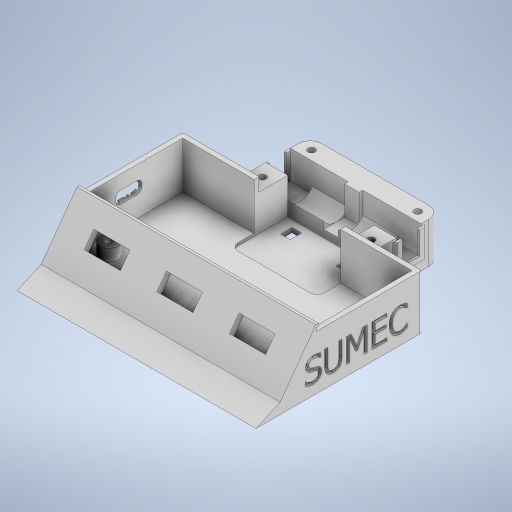
# Autodesk Inventor part: Sumec_telo_V4.1
Saved by Autodesk Inventor 2023 (Build 270158000, 158)
## iProperties
Created: 2023-03-18
Part Number: Sumec_telo_V4.1
Material: Všeobecné
Document SubType Name: Modeling
Designer: jaryj
Density: 1 g/cm^3
Appearance: Výchozí
Author: jaryj
Autodesk Inventor part; units mm, degrees
ref_plane "YZ Plane" through (0, 0, 0) normal (1, 0, 0) x (0, 1, 0)
ref_plane "XZ Plane" through (0, 0, 0) normal (0, 1, 0) x (-1, 0, 0)
ref_plane "XY Plane" through (0, 0, 0) normal (0, 0, 1) x (1, 0, 0)
sketch "Náčrt1" plane through (0, 0, 0) normal (0, 1, 0) x (-1, 0, 0)
  line L0 (0, 0) -> (49.75, 0)
  line L1 (49.75, 0) -> (49.75, -69)
  line L2 (49.75, -69) -> (18, -69)
  line L3 (18, -69) -> (18, -81)
  line L4 (18, -81) -> (27.25, -81)
  line L5 (27.25, -81) -> (27.25, -69)
  line L6 (27.25, -81) -> (27.25, -91.25)
  line L7 (27.25, -91.25) -> (27.25, -99.5)
  line L8 (27.25, -99.5) -> (0, -99.5)
  line L9 (0, -99.5) -> (0, -91.25)
  line L10 (0, -91.25) -> (27.25, -91.25)
  line L11 (0, -91.25) -> (0, -81)
  line L12 (0, -81) -> (18, -81)
  line L13 (0, -81) -> (0, 0)
  line L14 (18, -69) -> (18, -57.25)
  line L15 (18, -57.25) -> (0, -57.25)
  line L16 (47.75, -25) -> (47.75, -67)
  line L17 (47.75, -67) -> (18, -67)
  line L18 (0, -25) -> (47.75, -25)
  dimension "d0" = 49.75
  dimension "d1" = 69
  dimension "d2" = 12
  dimension "d3" = 10.25
  dimension "d4" = 8.25
  dimension "d5" = 27.25
  dimension "d6" = 18
  dimension "d9" = 2
  dimension "d13" = 25
  dimension "d18" = 2
  dimension "d190" = 9.75
  constraints: 38 end point, 12 perpendicular, 7 point on line, 1 horizontal, 1 vertical
  measures "d0" distance of L0.start L0.end
  measures "d1" distance of L0.end L1.end
  measures "d2" distance of L4.end L5.end
  measures "d3" distance of L4.end L6.end
  measures "d4" distance of L6.end L7.end
  measures "d5" distance of L7.end L8.end
  measures "d6" distance of L3.end L11.end
  measures "d9" distance between parallel lines of L17 L2
  measures "d13" distance between parallel lines of L0 L18
  measures "d18" distance between parallel lines of L1 L16
  measures "d190" distance between parallel lines of L17 L15
extrude "Vysunutí1" add sketch "Náčrt1" along normal blind 3 contours L18 L16 L17 L14 L15 L13
extrude "Vysunutí2" add sketch "Náčrt1" along normal blind 1.888 contours L15 L14 L3 L12 L13
extrude "Vysunutí3" add sketch "Náčrt1" along normal blind 22.5 contours L0 L1 L2 L14 L17 L16 L18 L13
extrude "Vysunutí4" add sketch "Náčrt1" along normal blind 17 contours L5 L4 L3 L2 | L10 L7 L8 L9
extrude "Vysunutí15" add sketch "Náčrt1" along normal blind 5 contours L12 L4 L6 L10 L11
sketch "Náčrt2" plane through (-49.75, 0, -69) normal (-1, 0, 0) x (0, 0, 1)
  line L0 (69, 0) -> (69, 22.5) projected
  line L1 (69, 0) -> (59, 4.5)
  line L2 (0, 0) -> (69, 0) projected
  line L3 (44, 0) -> (44, 22.5)
  line L4 (44, 3) -> (44, 22.5) projected
  line L5 (44, 22.5) -> (44, 25)
  line L6 (44, 25) -> (59, 4.5)
  line L7 (0, 22.5) -> (69, 22.5) projected
  point P0 (45.8293, 22.5)
  dimension "d23" = 25
  dimension "d24" = 4.5
  dimension "d25" = 10
  constraints: 8 end point, 2 point on line, 1 vertical
  measures "d23" distance of L3.start L5.end
  measures "d24" distance from line of L2 L1.end
  measures "d25" horizontal distance of L0.start L1.end
extrude "Vysunutí5" cut sketch "Náčrt2" against normal through all contours L1 L6 L7 L0
extrude "Vysunutí6" add sketch "Náčrt2" against normal up to surface (49.75 mm away) contours L7 L5 L6
sketch "Náčrt3" plane through (0, 3, -25) normal (0, 0, -1) x (-1, 0, 0)
  line L0 (22.75, 15.167) -> (37.75, 15.167)
  line L1 (37.75, 15.167) -> (37.75, 0)
  line L2 (37.75, 0) -> (22.75, 0)
  line L3 (22.75, 0) -> (22.75, 15.167)
  line L4 (0, 15.167) -> (7.5, 15.167)
  line L5 (7.5, 15.167) -> (7.5, 0)
  line L6 (7.5, 0) -> (0, 0)
  line L7 (0, 0) -> (0, 15.167)
  line L8 (49.75, -3) -> (0, -3) projected
  dimension "d30" = 15
  dimension "d31" = 7.5
  dimension "d32" = 15.167
  dimension "d33" = 3
  dimension "d34" = 15.25
  constraints: 16 end point, 4 perpendicular, 4 point on line, 1 horizontal, 1 vertical alignment
  measures "d30" distance of L0.start L0.end
  measures "d31" distance of L4.start L4.end
  measures "d32" distance of L0.end L1.end
  measures "d33" distance between parallel lines of L8 L6
  measures "d34" distance between parallel lines of L3 L5
extrude "Vysunutí7" cut sketch "Náčrt3" against normal blind 9
sketch "Náčrt7" plane through (-47.75, 3, -67) normal (1, 0, 0) x (0, 0, -1)
  line L0 (-57, 1.5) -> (-42, 22) projected
  line L1 (-42, 15.167) -> (-42, 0) projected
  line L2 (-42, 0) -> (-50, 0)
  line L3 (-42, 0) -> (-51, 0) projected
  line L4 (-50, 0) -> (-50, 6.833)
  line L5 (-50, 6.833) -> (-42, 17.7664)
  line L6 (-42, 17.7664) -> (-42, 0)
  point P0 (-67, -3)
  point P1 (-42, 22)
  point P2 (-38.3293, 19.5)
  point P3 (-36.5, 2)
  point P4 (-36.5, 2)
  dimension "d45" = 8
  dimension "d46" = 2.5
  constraints: 8 end point, 2 perpendicular, 1 collinear, 2 other
  measures "d45" distance of L2.start L2.end
extrude "Vysunutí9" cut sketch "Náčrt7" along normal through all
sketch "Náčrt13" plane through (0, 17, 0) normal (0, 1, 0) x (1, 0, 0)
  line L0 (-18, 81) -> (-27.25, 81) projected
  line L1 (-27.25, 81) -> (-27.25, 69) projected
  point P0 (0, 0)
  point P1 (-22.625, 75)
  dimension "d84" = 6
  dimension "d85" = 4.625
  measures "d84" distance from line of L0 point (-22.625, 75)
  measures "d85" distance from line of L1 point (-22.625, 75)
hole "Díra2" at (-22.625, 17, -75) direction (0, -1, 0) diameter 3 depth 6
sketch "Náčrt14" plane through (0, 17, 0) normal (0, 1, 0) x (1, 0, 0)
  line L0 (-27.25, 99.5) -> (-27.25, 91.25) projected
  line L1 (0, 99.5) -> (-27.25, 99.5) projected
  point P0 (0, 0)
  point P1 (-22.125, 95)
  dimension "d93" = 5.125
  dimension "d101" = 4.5
  measures "d93" distance from line of L0 point (-22.125, 95)
  measures "d101" distance from line of L1 point (-22.125, 95)
hole "Díra3" at (-22.125, 17, -95) direction (0, -1, 0) diameter 3 depth 6
fillet "Zaoblení1" radius 3 1 edges at (-18, 2.444, -57.25)
fillet "Zaoblení2" radius 1 1 edges at (-49.75, 11.25, -69)
fillet "Zaoblení3" radius 5 1 edges at (-27.25, 8.5, -99.5)
sketch "Náčrt24" plane through (-18, 3, -67) normal (1, 0, 0) x (0, 0, -1)
  line L0 (24.25, 2) -> (24.25, 14) projected
  line L1 (24.25, 2) -> (14, 2) projected
  line L2 (14, 2) -> (14, 14) projected
  line L3 (14, 2) -> (24.25, 2) projected
  line L4 (24.25, 4.88) -> (24.25, 2)
  line L5 (24.25, 2) -> (14, 2)
  line L6 (14, 2) -> (14, 4.88)
  arc A0 (14, 4.88) -> (24.25, 4.88) centre (19.125, 8) ccw
  point P0 (-67, -3)
  point P1 (19.125, 2)
  dimension "d200" = 6
  constraints: 6 end point, 2 perpendicular, 2 point on circle, 2 point on line, 1 centre point, 1 horizontal alignment, 1 tangent
  measures "d200" radius of A0
extrude "Vysunutí22" add sketch "Náčrt24" along normal blind 15
sketch "Náčrt21" plane through (-27.25, 0, -69) normal (-1, 0, 0) x (0, 0, 1)
  line L0 (-20.75, 16) -> (-23.75, 16)
  line L1 (-22.25, 17) -> (-30.5, 17) projected
  line L2 (-23.75, 3.5) -> (-10.5, 3.5)
  line L3 (-10.5, 3.5) -> (-10.5, 16)
  line L4 (-10.5, 16) -> (-13.5, 16)
  line L5 (-13.5, 16) -> (-13.5, 6.5)
  line L6 (-13.5, 6.5) -> (-20.75, 6.5)
  line L7 (-20.75, 6.5) -> (-20.75, 16)
  line L8 (-23.75, 16) -> (-23.75, 3.5)
  line L9 (-22.25, 5) -> (-22.25, 17) projected
  line L10 (-22.25, 5) -> (-12, 5) projected
  line L11 (-12, 5) -> (-12, 17) projected
  line L12 (-12, 17) -> (0, 17) projected
  point P0 (69, 0)
  dimension "d172" = 1.5
  dimension "d173" = 1.5
  dimension "d174" = 1.5
  dimension "d175" = 1.5
  dimension "d176" = 1.5
  dimension "d177" = 1.5
  dimension "d180" = 1
  constraints: 12 end point, 3 perpendicular, 1 horizontal, 1 parallel, 1 vertical, 8 other
  measures "d172" distance between parallel lines of L7 L9
  measures "d173" distance between parallel lines of L6 L10
  measures "d174" distance between parallel lines of L5 L11
  measures "d175" distance between parallel lines of L11 L3
  measures "d176" distance between parallel lines of L2 L10
  measures "d177" distance between parallel lines of L8 L9
extrude "Vysunutí19" add sketch "Náčrt21" along normal blind 1
chamfer "Zkosení1" distance 1 angle 45 3 edges at (-28.25, 9.75, -92.75) (-28.25, 3.5, -86.125) (-28.25, 9.75, -79.5)
sketch "Náčrt27" plane through (-49.75, 22.5, -25) normal (-1, 0, 0) x (0, 0, 1)
  line L0 (0, 2.5) -> (0, 0) projected
  line L1 (0, 2.5) -> (-1, 2.5)
  line L2 (-1, 2.5) -> (-1, 1.5)
  line L3 (-1, 1.5) -> (0, 1.5)
  line L4 (0, 1.5) -> (0, 2.5)
  point P0 (25, -22.5)
  point P1 (0, 1.5)
  dimension "d219" = 1
  dimension "d220" = 1
  constraints: 8 end point, 2 parallel, 1 horizontal, 1 perpendicular
  measures "d219" distance of L2.end L3.end
  measures "d220" distance of L1.end L2.end
extrude "Vysunutí25" add sketch "Náčrt27" against normal up to surface (49.75 mm away)
mirror "Zrcadlit1" about plane through (0, 0, -25) normal (1, 0, 0)
sketch "Náčrt16" plane through (0, 1.888, 0) normal (0, 1, 0) x (1, 0, 0)
  line L0 (-9.4, 73.375) -> (-13.4, 73.375)
  line L1 (-13.4, 73.375) -> (-13.4, 78.125)
  line L2 (-13.4, 78.125) -> (-9.4, 78.125)
  line L3 (-9.4, 78.125) -> (-9.4, 73.375)
  line L4 (-18, 69) -> (-18, 81) projected
  line L5 (13.75, 73.375) -> (9.75, 73.375)
  line L6 (9.75, 73.375) -> (9.75, 78.125)
  line L7 (9.75, 78.125) -> (13.75, 78.125)
  line L8 (13.75, 78.125) -> (13.75, 73.375)
  line L9 (18, 69) -> (18, 81) projected
  line L10 (-18, 81) -> (18, 81) projected
  point P0 (0, 0)
  dimension "d128" = 4
  dimension "d129" = 4.75
  dimension "d130" = 4.6
  dimension "d134" = 4.25
  dimension "d192" = 2.875
  constraints: 16 end point, 4 parallel, 2 equal length, 2 perpendicular, 1 horizontal, 1 horizontal alignment
  measures "d128" distance of L0.start L0.end
  measures "d129" distance of L2.end L0.start
  measures "d130" distance between parallel lines of L4 L1
  measures "d134" distance between parallel lines of L9 L8
  measures "d192" distance between parallel lines of L10 L2
extrude "Vysunutí16" cut sketch "Náčrt16" against normal through all
sketch "Náčrt17" plane through (0, 3, 0) normal (0, 1, 0) x (1, 0, 0)
  line L0 (-47.75, 17) -> (-37.75, 17) projected
  line L1 (-47.75, 17) -> (-47.75, 67) projected
  line L2 (47.75, 17) -> (37.75, 17) projected
  line L3 (47.75, 17) -> (47.75, 67) projected
  line L4 (-39.4, 19.625) -> (-43.4, 19.625)
  line L5 (-43.4, 19.625) -> (-43.4, 24.375)
  line L6 (-43.4, 24.375) -> (-39.4, 24.375)
  line L7 (-39.4, 24.375) -> (-39.4, 19.625)
  line L8 (42.75, 19.625) -> (38.75, 19.625)
  line L9 (38.75, 19.625) -> (38.75, 24.375)
  line L10 (38.75, 24.375) -> (42.75, 24.375)
  line L11 (42.75, 24.375) -> (42.75, 19.625)
  point P0 (0, 0)
  point P1 (-48, 67)
  point P2 (48, 67)
  point P3 (-41.4, 19.625)
  point P4 (40.75, 19.625)
  point P5 (-47.75, 67)
  point P6 (47.75, 67)
  dimension "d137" = 4
  dimension "d138" = 4.75
  dimension "d139" = 4.35
  dimension "d143" = 2.625
  dimension "d144" = 5
  dimension "d146" = 2.625
  constraints: 16 end point, 4 parallel, 2 equal length, 2 horizontal, 2 midpoint, 2 perpendicular, 2 other
  measures "d137" distance of L4.start L4.end
  measures "d138" distance of L6.end L4.start
  measures "d143" distance between parallel lines of L0 L4
  measures "d146" distance from line of L2 point (40.75, 19.625)
extrude "Vysunutí17" cut sketch "Náčrt17" against normal through all
sketch "Náčrt18" plane through (0, 3, 0) normal (0, 1, 0) x (1, 0, 0)
  circle A0 centre (39.25, 59) radius 3.75
  circle A1 centre (-40.5, 29) radius 3.75
  line L0 (47.75, 67) -> (18, 67) projected
  line L1 (47.75, 25) -> (47.75, 67) projected
  line L2 (-47.75, 17) -> (-37.75, 17) projected
  line L3 (-47.75, 17) -> (-47.75, 67) projected
  point P0 (0, 0)
  point P1 (42.5, 67)
  point P2 (-48, 67)
  point P3 (-47.75, 67)
  dimension "d149" = 7.5
  dimension "d150" = 8
  dimension "d151" = 8.5
  dimension "d152" = 12
  dimension "d153" = 7.25
  constraints: 2 centre point, 1 equal radius, 1 other
  measures "d149" diameter of A0
  measures "d150" distance from line of A0.centre L0
  measures "d151" distance from line of L1 A0.centre
  measures "d152" distance from line of L2 A1.centre
extrude "Vysunutí18" add sketch "Náčrt18" along normal blind 5
sketch "Náčrt19" plane through (39.25, 8, -59) normal (0, 1, 0) x (1, 0, 0)
  circle A0 centre (0, 0) radius 3.75 projected
  point P0 (-39.25, -59)
  constraints: 1 coincident
hole "Díra4" at (39.25, 8, -59) direction (0, -1, 0) diameter 3 depth 6
sketch "Náčrt20" plane through (-40.5, 8, -29) normal (0, 1, 0) x (1, 0, 0)
  circle A0 centre (0, 0) radius 3.75 projected
  point P0 (40.5, -29)
  constraints: 1 coincident
hole "Díra5" at (-40.5, 8, -29) direction (0, -1, 0) diameter 3 depth 6
sketch "Náčrt25" plane through (-18, 7.88, -91.25) normal (0, 0, 1) x (1, 0, 0)
  line L0 (-4.25, 9.12) -> (40.25, 9.12) projected
  line L1 (15, 9.12) -> (21, 9.12)
  line L2 (21, 9.12) -> (21, -2.88)
  line L3 (21, -2.88) -> (15, -2.88)
  line L4 (15, -2.88) -> (15, 9.12)
  line L5 (15, 0) -> (15, -2.88) projected
  line L6 (21, 0) -> (21, -2.88) projected
  point P0 (18, -7.88)
  dimension "d203" = 12
  dimension "d204" = 6
  constraints: 8 end point, 2 parallel, 1 coincident, 1 horizontal, 1 perpendicular, 1 point on line
  measures "d203" distance of L3.end L1.start
  measures "d204" distance between parallel lines of L2 L4
extrude "Vysunutí23" add sketch "Náčrt25" along normal blind 1.5
sketch "Náčrt26" plane through (-49.75, 0, -68) normal (-1, 0, 0) x (0, 0, 1)
  line L0 (20, 11.7) -> (27, 11.7)
  line L1 (27, 16.7) -> (20, 16.7)
  line L2 (18, 14.7) -> (18, 13.7)
  line L3 (29, 14.7) -> (29, 13.7)
  line L4 (0, 0) -> (68, 0) projected
  line L5 (0, 0) -> (0, 22.5) projected
  arc A0 (20, 16.7) -> (18, 14.7) centre (20, 14.7) ccw
  arc A1 (18, 13.7) -> (20, 11.7) centre (20, 13.7) ccw
  arc A2 (29, 14.7) -> (27, 16.7) centre (27, 14.7) ccw
  arc A3 (27, 11.7) -> (29, 13.7) centre (27, 13.7) ccw
  dimension "d207" = 11.7
  dimension "d208" = 5
  dimension "d209" = 11
  dimension "d210" = 18
  dimension "d211" = 2
  constraints: 8 end point, 8 point on circle, 8 tangent, 4 centre point, 3 equal radius, 1 horizontal, 1 parallel, 1 vertical
  measures "d207" distance between parallel lines of L4 L0
  measures "d208" distance between parallel lines of L0 L1
  measures "d209" distance between parallel lines of L3 L2
  measures "d210" distance between parallel lines of L5 L2
  measures "d211" radius of A0
extrude "Vysunutí24" cut sketch "Náčrt26" against normal up to surface (2 mm away)
sketch "Náčrt28" plane through (49.75, 0, 0) normal (1, 0, 0) x (0, 0, -1)
  line L0 (20, 14.5) -> (64, 14.5) construction
  line L1 (64, 14.5) -> (64, 4) construction
  line L2 (64, 4) -> (20, 4) construction
  line L3 (20, 4) -> (20, 14.5) construction
  line L4 (68, 22.5) -> (25, 22.5) projected
  line L5 (68, 0) -> (68, 22.5) projected
  spline S0 degree 2 poles (23.8006, 4.1434) (22.7147, 4.1434) (21.1912, 4.5972) (20.5186, 4.9214) knots 0 0 0 1 2 2 2
  line L6 (20.5186, 4.9214) -> (20.5186, 6.5908)
  line L7 (20.5186, 6.5908) -> (20.6159, 6.5908)
  spline S1 degree 2 poles (20.6159, 6.5908) (21.2723, 5.9749) (22.9335, 5.2942) (23.7034, 5.2942) knots 0 0 0 1 2 2 2
  spline S2 degree 2 poles (23.7034, 5.2942) (24.8055, 5.2942) (25.9319, 6.2099) (25.9319, 6.9635) knots 0 0 0 1 2 2 2
  spline S3 degree 2 poles (25.9319, 6.9635) (25.9319, 7.5632) (25.3404, 8.3088) (24.7002, 8.4951) knots 0 0 0 1 2 2 2
  spline S4 degree 2 poles (24.7002, 8.4951) (24.2382, 8.6248) (23.4684, 8.8031) (22.893, 8.9489) knots 0 0 0 1 2 2 2
  spline S5 degree 2 poles (22.893, 8.9489) (22.3744, 9.0867) (21.5559, 9.5) (21.2399, 9.8323) knots 0 0 0 1 2 2 2
  spline S6 degree 2 poles (21.2399, 9.8323) (20.9319, 10.1645) (20.5916, 11.0559) (20.5916, 11.6394) knots 0 0 0 1 2 2 2
  spline S7 degree 2 poles (20.5916, 11.6394) (20.5916, 12.8549) (22.4878, 14.5) (23.9546, 14.5) knots 0 0 0 1 2 2 2
  spline S8 degree 2 poles (23.9546, 14.5) (24.7974, 14.5) (26.2885, 14.1677) (26.9287, 13.8517) knots 0 0 0 1 2 2 2
  line L8 (26.9287, 13.8517) -> (26.9287, 12.2634)
  line L9 (26.9287, 12.2634) -> (26.8314, 12.2634)
  spline S9 degree 2 poles (26.8314, 12.2634) (26.3533, 12.701) (24.8622, 13.3493) (24.0438, 13.3493) knots 0 0 0 1 2 2 2
  spline S10 degree 2 poles (24.0438, 13.3493) (23.1199, 13.3493) (21.9773, 12.4822) (21.9773, 11.7771) knots 0 0 0 1 2 2 2
  spline S11 degree 2 poles (21.9773, 11.7771) (21.9773, 11.1451) (22.6499, 10.3914) (23.282, 10.2212) knots 0 0 0 1 2 2 2
  spline S12 degree 2 poles (23.282, 10.2212) (23.7034, 10.1078) (24.9271, 9.816) (25.3323, 9.6945) knots 0 0 0 1 2 2 2
  spline S13 degree 2 poles (25.3323, 9.6945) (26.3614, 9.3784) (27.3177, 8.1062) (27.3177, 7.1742) knots 0 0 0 1 2 2 2
  spline S14 degree 2 poles (27.3177, 7.1742) (27.3177, 6.5827) (26.8395, 5.4481) (26.41, 5.0511) knots 0 0 0 1 2 2 2
  spline S15 degree 2 poles (26.41, 5.0511) (25.9319, 4.6135) (24.7164, 4.1434) (23.8006, 4.1434) knots 0 0 0 1 2 2 2
  spline S16 degree 2 poles (32.1637, 4.111) (31.2804, 4.111) (29.9676, 4.5729) (29.5057, 5.0348) knots 0 0 0 1 2 2 2
  spline S17 degree 2 poles (29.5057, 5.0348) (28.9789, 5.5535) (28.5494, 7.0122) (28.5494, 8.0818) knots 0 0 0 1 2 2 2
  line L10 (28.5494, 8.0818) -> (28.5494, 14.3217)
  line L11 (28.5494, 14.3217) -> (29.8784, 14.3217)
  line L12 (29.8784, 14.3217) -> (29.8784, 8.0818)
  spline S18 degree 2 poles (29.8784, 8.0818) (29.8784, 7.3849) (30.0567, 6.4449) (30.3079, 6.064) knots 0 0 0 1 2 2 2
  spline S19 degree 2 poles (30.3079, 6.064) (30.5754, 5.6588) (31.4992, 5.2455) (32.1637, 5.2455) knots 0 0 0 1 2 2 2
  spline S20 degree 2 poles (32.1637, 5.2455) (32.7877, 5.2455) (33.7601, 5.6588) (34.0276, 6.064) knots 0 0 0 1 2 2 2
  spline S21 degree 2 poles (34.0276, 6.064) (34.2788, 6.4449) (34.4571, 7.3768) (34.4571, 8.0494) knots 0 0 0 1 2 2 2
  line L13 (34.4571, 8.0494) -> (34.4571, 14.3217)
  line L14 (34.4571, 14.3217) -> (35.7861, 14.3217)
  line L15 (35.7861, 14.3217) -> (35.7861, 8.0818)
  spline S22 degree 2 poles (35.7861, 8.0818) (35.7861, 7.0365) (35.3647, 5.5454) (34.8298, 5.0348) knots 0 0 0 1 2 2 2
  spline S23 degree 2 poles (34.8298, 5.0348) (34.3517, 4.5648) (33.0875, 4.111) (32.1637, 4.111) knots 0 0 0 1 2 2 2
  line L16 (46.2642, 4.3217) -> (44.9352, 4.3217)
  line L17 (44.9352, 4.3217) -> (44.9352, 12.936)
  line L18 (44.9352, 12.936) -> (42.3258, 7.077)
  line L19 (42.3258, 7.077) -> (41.5154, 7.077)
  line L20 (41.5154, 7.077) -> (38.9303, 12.936)
  line L21 (38.9303, 12.936) -> (38.9303, 4.3217)
  line L22 (38.9303, 4.3217) -> (37.6904, 4.3217)
  line L23 (37.6904, 4.3217) -> (37.6904, 14.3217)
  line L24 (37.6904, 14.3217) -> (39.5057, 14.3217)
  line L25 (39.5057, 14.3217) -> (42.0016, 8.7545)
  line L26 (42.0016, 8.7545) -> (44.4165, 14.3217)
  line L27 (44.4165, 14.3217) -> (46.2642, 14.3217)
  line L28 (46.2642, 14.3217) -> (46.2642, 4.3217)
  line L29 (48.2901, 4.3217) -> (48.2901, 14.3217)
  line L30 (48.2901, 14.3217) -> (54.5462, 14.3217)
  line L31 (54.5462, 14.3217) -> (54.5462, 13.1386)
  line L32 (54.5462, 13.1386) -> (49.6191, 13.1386)
  line L33 (49.6191, 13.1386) -> (49.6191, 10.3995)
  line L34 (49.6191, 10.3995) -> (54.2139, 10.3995)
  line L35 (54.2139, 10.3995) -> (54.2139, 9.2164)
  line L36 (54.2139, 9.2164) -> (49.6191, 9.2164)
  line L37 (49.6191, 9.2164) -> (49.6191, 5.5049)
  line L38 (49.6191, 5.5049) -> (54.5462, 5.5049)
  line L39 (54.5462, 5.5049) -> (54.5462, 4.3217)
  line L40 (54.5462, 4.3217) -> (48.2901, 4.3217)
  spline S24 degree 2 poles (59.9109, 4.1434) (58.9384, 4.1434) (57.2934, 4.7998) (56.6937, 5.4562) knots 0 0 0 1 2 2 2
  spline S25 degree 2 poles (56.6937, 5.4562) (56.094, 6.1045) (55.4376, 8.0494) (55.4376, 9.3136) knots 0 0 0 1 2 2 2
  spline S26 degree 2 poles (55.4376, 9.3136) (55.4376, 10.5697) (56.0778, 12.4335) (56.6856, 13.1224) knots 0 0 0 1 2 2 2
  spline S27 degree 2 poles (56.6856, 13.1224) (57.2853, 13.795) (58.9222, 14.5) (59.9352, 14.5) knots 0 0 0 1 2 2 2
  spline S28 degree 2 poles (59.9352, 14.5) (60.4376, 14.5) (61.3209, 14.3541) (61.6937, 14.2407) knots 0 0 0 1 2 2 2
  spline S29 degree 2 poles (61.6937, 14.2407) (62.0178, 14.1353) (62.6904, 13.8355) (63.0227, 13.6572) knots 0 0 0 1 2 2 2
  line L41 (63.0227, 13.6572) -> (63.0227, 12.0527)
  line L42 (63.0227, 12.0527) -> (62.9173, 12.0527)
  spline S30 degree 2 poles (62.9173, 12.0527) (62.7391, 12.2147) (62.188, 12.6686) (61.7909, 12.8874) knots 0 0 0 1 2 2 2
  spline S31 degree 2 poles (61.7909, 12.8874) (61.41, 13.0981) (60.5105, 13.3655) (59.9271, 13.3655) knots 0 0 0 1 2 2 2
  spline S32 degree 2 poles (59.9271, 13.3655) (59.2869, 13.3655) (58.1442, 12.8387) (57.7147, 12.3363) knots 0 0 0 1 2 2 2
  spline S33 degree 2 poles (57.7147, 12.3363) (57.2934, 11.8258) (56.8233, 10.278) (56.8233, 9.3136) knots 0 0 0 1 2 2 2
  spline S34 degree 2 poles (56.8233, 9.3136) (56.8233, 8.2844) (57.3177, 6.8015) (57.7472, 6.2909) knots 0 0 0 1 2 2 2
  spline S35 degree 2 poles (57.7472, 6.2909) (58.1686, 5.7966) (59.295, 5.2942) (59.9271, 5.2942) knots 0 0 0 1 2 2 2
  spline S36 degree 2 poles (59.9271, 5.2942) (60.5024, 5.2942) (61.483, 5.5778) (61.8639, 5.7885) knots 0 0 0 1 2 2 2
  spline S37 degree 2 poles (61.8639, 5.7885) (62.2285, 5.9992) (62.7715, 6.4368) (62.9254, 6.5908) knots 0 0 0 1 2 2 2
  line L43 (62.9254, 6.5908) -> (63.0227, 6.5908)
  line L44 (63.0227, 6.5908) -> (63.0227, 5.0024)
  spline S38 degree 2 poles (63.0227, 5.0024) (62.6904, 4.8485) (62.107, 4.5648) (61.6937, 4.4352) knots 0 0 0 1 2 2 2
  spline S39 degree 2 poles (61.6937, 4.4352) (61.2561, 4.2893) (60.5105, 4.1434) (59.9109, 4.1434) knots 0 0 0 1 2 2 2
  point P0 (0, 0)
  dimension "d229" = 8
  dimension "d230" = 4
  dimension "d231" = 44
  dimension "d232" = 10.5
  constraints: 2 other
  measures "d229" distance between parallel lines of L4 L0
  measures "d230" distance between parallel lines of L5 L1
  measures "d231" distance of L0.start L0.end
  measures "d232" distance of L2.end L0.start
extrude "Vysunutí26" cut sketch "Náčrt28" against normal blind 1
sketch "Náčrt29" plane through (-49.75, 0, -68) normal (-1, 0, 0) x (0, 0, 1)
  line L0 (3, 14.5) -> (47, 14.5) construction
  line L1 (47, 14.5) -> (47, 4) construction
  line L2 (47, 4) -> (3, 4) construction
  line L3 (3, 4) -> (3, 14.5) construction
  line L4 (0, 22.5) -> (43, 22.5) projected
  line L5 (-1, 22.5) -> (-1, 0) projected
  spline S0 degree 2 poles (6.8006, 4.1434) (5.7147, 4.1434) (4.1912, 4.5972) (3.5186, 4.9214) knots 0 0 0 1 2 2 2
  line L6 (3.5186, 4.9214) -> (3.5186, 6.5908)
  line L7 (3.5186, 6.5908) -> (3.6159, 6.5908)
  spline S1 degree 2 poles (3.6159, 6.5908) (4.2723, 5.9749) (5.9335, 5.2942) (6.7034, 5.2942) knots 0 0 0 1 2 2 2
  spline S2 degree 2 poles (6.7034, 5.2942) (7.8055, 5.2942) (8.9319, 6.2099) (8.9319, 6.9635) knots 0 0 0 1 2 2 2
  spline S3 degree 2 poles (8.9319, 6.9635) (8.9319, 7.5632) (8.3404, 8.3088) (7.7002, 8.4951) knots 0 0 0 1 2 2 2
  spline S4 degree 2 poles (7.7002, 8.4951) (7.2382, 8.6248) (6.4684, 8.8031) (5.893, 8.9489) knots 0 0 0 1 2 2 2
  spline S5 degree 2 poles (5.893, 8.9489) (5.3744, 9.0867) (4.5559, 9.5) (4.2399, 9.8323) knots 0 0 0 1 2 2 2
  spline S6 degree 2 poles (4.2399, 9.8323) (3.9319, 10.1645) (3.5916, 11.0559) (3.5916, 11.6394) knots 0 0 0 1 2 2 2
  spline S7 degree 2 poles (3.5916, 11.6394) (3.5916, 12.8549) (5.4878, 14.5) (6.9546, 14.5) knots 0 0 0 1 2 2 2
  spline S8 degree 2 poles (6.9546, 14.5) (7.7974, 14.5) (9.2885, 14.1677) (9.9287, 13.8517) knots 0 0 0 1 2 2 2
  line L8 (9.9287, 13.8517) -> (9.9287, 12.2634)
  line L9 (9.9287, 12.2634) -> (9.8314, 12.2634)
  spline S9 degree 2 poles (9.8314, 12.2634) (9.3533, 12.701) (7.8622, 13.3493) (7.0438, 13.3493) knots 0 0 0 1 2 2 2
  spline S10 degree 2 poles (7.0438, 13.3493) (6.1199, 13.3493) (4.9773, 12.4822) (4.9773, 11.7771) knots 0 0 0 1 2 2 2
  spline S11 degree 2 poles (4.9773, 11.7771) (4.9773, 11.1451) (5.6499, 10.3914) (6.282, 10.2212) knots 0 0 0 1 2 2 2
  spline S12 degree 2 poles (6.282, 10.2212) (6.7034, 10.1078) (7.9271, 9.816) (8.3323, 9.6945) knots 0 0 0 1 2 2 2
  spline S13 degree 2 poles (8.3323, 9.6945) (9.3614, 9.3784) (10.3177, 8.1062) (10.3177, 7.1742) knots 0 0 0 1 2 2 2
  spline S14 degree 2 poles (10.3177, 7.1742) (10.3177, 6.5827) (9.8395, 5.4481) (9.41, 5.0511) knots 0 0 0 1 2 2 2
  spline S15 degree 2 poles (9.41, 5.0511) (8.9319, 4.6135) (7.7164, 4.1434) (6.8006, 4.1434) knots 0 0 0 1 2 2 2
  spline S16 degree 2 poles (15.1637, 4.111) (14.2804, 4.111) (12.9676, 4.5729) (12.5057, 5.0348) knots 0 0 0 1 2 2 2
  spline S17 degree 2 poles (12.5057, 5.0348) (11.9789, 5.5535) (11.5494, 7.0122) (11.5494, 8.0818) knots 0 0 0 1 2 2 2
  line L10 (11.5494, 8.0818) -> (11.5494, 14.3217)
  line L11 (11.5494, 14.3217) -> (12.8784, 14.3217)
  line L12 (12.8784, 14.3217) -> (12.8784, 8.0818)
  spline S18 degree 2 poles (12.8784, 8.0818) (12.8784, 7.3849) (13.0567, 6.4449) (13.3079, 6.064) knots 0 0 0 1 2 2 2
  spline S19 degree 2 poles (13.3079, 6.064) (13.5754, 5.6588) (14.4992, 5.2455) (15.1637, 5.2455) knots 0 0 0 1 2 2 2
  spline S20 degree 2 poles (15.1637, 5.2455) (15.7877, 5.2455) (16.7601, 5.6588) (17.0276, 6.064) knots 0 0 0 1 2 2 2
  spline S21 degree 2 poles (17.0276, 6.064) (17.2788, 6.4449) (17.4571, 7.3768) (17.4571, 8.0494) knots 0 0 0 1 2 2 2
  line L13 (17.4571, 8.0494) -> (17.4571, 14.3217)
  line L14 (17.4571, 14.3217) -> (18.7861, 14.3217)
  line L15 (18.7861, 14.3217) -> (18.7861, 8.0818)
  spline S22 degree 2 poles (18.7861, 8.0818) (18.7861, 7.0365) (18.3647, 5.5454) (17.8298, 5.0348) knots 0 0 0 1 2 2 2
  spline S23 degree 2 poles (17.8298, 5.0348) (17.3517, 4.5648) (16.0875, 4.111) (15.1637, 4.111) knots 0 0 0 1 2 2 2
  line L16 (29.2642, 4.3217) -> (27.9352, 4.3217)
  line L17 (27.9352, 4.3217) -> (27.9352, 12.936)
  line L18 (27.9352, 12.936) -> (25.3258, 7.077)
  line L19 (25.3258, 7.077) -> (24.5154, 7.077)
  line L20 (24.5154, 7.077) -> (21.9303, 12.936)
  line L21 (21.9303, 12.936) -> (21.9303, 4.3217)
  line L22 (21.9303, 4.3217) -> (20.6904, 4.3217)
  line L23 (20.6904, 4.3217) -> (20.6904, 14.3217)
  line L24 (20.6904, 14.3217) -> (22.5057, 14.3217)
  line L25 (22.5057, 14.3217) -> (25.0016, 8.7545)
  line L26 (25.0016, 8.7545) -> (27.4165, 14.3217)
  line L27 (27.4165, 14.3217) -> (29.2642, 14.3217)
  line L28 (29.2642, 14.3217) -> (29.2642, 4.3217)
  line L29 (31.2901, 4.3217) -> (31.2901, 14.3217)
  line L30 (31.2901, 14.3217) -> (37.5462, 14.3217)
  line L31 (37.5462, 14.3217) -> (37.5462, 13.1386)
  line L32 (37.5462, 13.1386) -> (32.6191, 13.1386)
  line L33 (32.6191, 13.1386) -> (32.6191, 10.3995)
  line L34 (32.6191, 10.3995) -> (37.2139, 10.3995)
  line L35 (37.2139, 10.3995) -> (37.2139, 9.2164)
  line L36 (37.2139, 9.2164) -> (32.6191, 9.2164)
  line L37 (32.6191, 9.2164) -> (32.6191, 5.5049)
  line L38 (32.6191, 5.5049) -> (37.5462, 5.5049)
  line L39 (37.5462, 5.5049) -> (37.5462, 4.3217)
  line L40 (37.5462, 4.3217) -> (31.2901, 4.3217)
  spline S24 degree 2 poles (42.9109, 4.1434) (41.9384, 4.1434) (40.2934, 4.7998) (39.6937, 5.4562) knots 0 0 0 1 2 2 2
  spline S25 degree 2 poles (39.6937, 5.4562) (39.094, 6.1045) (38.4376, 8.0494) (38.4376, 9.3136) knots 0 0 0 1 2 2 2
  spline S26 degree 2 poles (38.4376, 9.3136) (38.4376, 10.5697) (39.0778, 12.4335) (39.6856, 13.1224) knots 0 0 0 1 2 2 2
  spline S27 degree 2 poles (39.6856, 13.1224) (40.2853, 13.795) (41.9222, 14.5) (42.9352, 14.5) knots 0 0 0 1 2 2 2
  spline S28 degree 2 poles (42.9352, 14.5) (43.4376, 14.5) (44.3209, 14.3541) (44.6937, 14.2407) knots 0 0 0 1 2 2 2
  spline S29 degree 2 poles (44.6937, 14.2407) (45.0178, 14.1353) (45.6904, 13.8355) (46.0227, 13.6572) knots 0 0 0 1 2 2 2
  line L41 (46.0227, 13.6572) -> (46.0227, 12.0527)
  line L42 (46.0227, 12.0527) -> (45.9173, 12.0527)
  spline S30 degree 2 poles (45.9173, 12.0527) (45.7391, 12.2147) (45.188, 12.6686) (44.7909, 12.8874) knots 0 0 0 1 2 2 2
  spline S31 degree 2 poles (44.7909, 12.8874) (44.41, 13.0981) (43.5105, 13.3655) (42.9271, 13.3655) knots 0 0 0 1 2 2 2
  spline S32 degree 2 poles (42.9271, 13.3655) (42.2869, 13.3655) (41.1442, 12.8387) (40.7147, 12.3363) knots 0 0 0 1 2 2 2
  spline S33 degree 2 poles (40.7147, 12.3363) (40.2934, 11.8258) (39.8233, 10.278) (39.8233, 9.3136) knots 0 0 0 1 2 2 2
  spline S34 degree 2 poles (39.8233, 9.3136) (39.8233, 8.2844) (40.3177, 6.8015) (40.7472, 6.2909) knots 0 0 0 1 2 2 2
  spline S35 degree 2 poles (40.7472, 6.2909) (41.1686, 5.7966) (42.295, 5.2942) (42.9271, 5.2942) knots 0 0 0 1 2 2 2
  spline S36 degree 2 poles (42.9271, 5.2942) (43.5024, 5.2942) (44.483, 5.5778) (44.8639, 5.7885) knots 0 0 0 1 2 2 2
  spline S37 degree 2 poles (44.8639, 5.7885) (45.2285, 5.9992) (45.7715, 6.4368) (45.9254, 6.5908) knots 0 0 0 1 2 2 2
  line L43 (45.9254, 6.5908) -> (46.0227, 6.5908)
  line L44 (46.0227, 6.5908) -> (46.0227, 5.0024)
  spline S38 degree 2 poles (46.0227, 5.0024) (45.6904, 4.8485) (45.107, 4.5648) (44.6937, 4.4352) knots 0 0 0 1 2 2 2
  spline S39 degree 2 poles (44.6937, 4.4352) (44.2561, 4.2893) (43.5105, 4.1434) (42.9109, 4.1434) knots 0 0 0 1 2 2 2
  point P0 (68, 0)
  dimension "d225" = 8
  dimension "d226" = 4
  dimension "d233" = 44
  dimension "d234" = 10.5
  constraints: 2 other
  measures "d225" distance between parallel lines of L4 L0
  measures "d226" distance between parallel lines of L5 L3
  measures "d233" distance of L0.start L0.end
  measures "d234" distance of L0.end L1.end
extrude "Vysunutí27" cut sketch "Náčrt29" against normal blind 1
